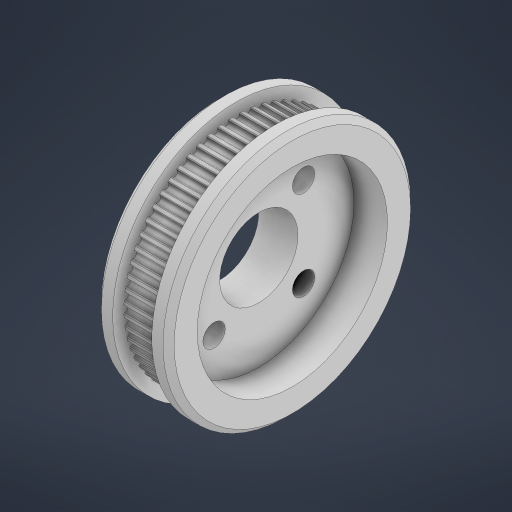
# Autodesk Inventor part: GT2 Pulley
Saved by Autodesk Inventor 2024 (Build 280153000, 153)
## iProperties
Created: 2023-10-25
Part Number: GT2 Pulley
Material: Generic
Document SubType Name: Modeling
Designer: avsar
Density: 1 g/cm^3
Appearance: Default
Author: avsar
Autodesk Inventor part; units mm, degrees
ref_plane "YZ Plane" through (0, 0, 0) normal (1, 0, 0) x (0, 1, 0)
ref_plane "XZ Plane" through (0, 0, 0) normal (0, 1, 0) x (-1, 0, 0)
ref_plane "XY Plane" through (0, 0, 0) normal (0, 0, 1) x (1, 0, 0)
sketch "Sketch1" plane through (0, 0, 0) normal (1, 0, 0) x (0, 1, 0)
  circle A0 centre (0, 0) radius 20.1178 construction
  circle A1 centre (0, 0) radius 19.3678 construction
  line L0 (0, 0) -> (20.1178, 0) construction
  line L1 (0, 0) -> (0, -20.1178) construction
  circle A2 centre (19.9228, 0) radius 0.555 construction
  line L2 (0, 0) -> (20.021, -1.9719) construction
  circle A3 centre (19.8269, -1.9528) radius 0.555 construction
  circle A4 centre (19.9554, -0.7042) radius 0.15 construction
  circle A5 centre (19.9283, -1.2551) radius 0.15 construction
  arc A6 (19.3678, 0) -> (19.9485, -0.5544) centre (19.9228, 0) ccw
  arc A7 (20.1053, -0.7095) -> (19.9485, -0.5544) centre (19.9554, -0.7042) ccw
  arc A8 (20.0781, -1.2645) -> (20.1053, -0.7095) centre (0, 0) ccw
  arc A9 (19.9068, -1.4036) -> (20.0781, -1.2645) centre (19.9283, -1.2551) ccw
  arc A10 (19.9068, -1.4036) -> (19.2746, -1.8984) centre (19.8269, -1.9528) ccw
  arc A11 (19.2746, -1.8984) -> (19.3678, 0) centre (0, 0) ccw
  dimension "d0" = 40.2357
  dimension "d1" = -0.75
  dimension "d2" = 1.11
  dimension "d4" = 84.375
  dimension "d5" = 0.3
  constraints: 25 point on circle, 12 centre point, 8 equal radius, 8 tangent, 6 end point, 4 point on line, 1 coincident, 1 concentric, 1 horizontal, 1 perpendicular
  measures "d0" diameter of A0
  measures "d1" radial gap between concentric circles of A0 A1
  measures "d2" diameter of A2
  measures "d4" angle of L1 L2
  measures "d5" diameter of A4
extrude "Extrusion1" add sketch "Sketch1" along normal mid plane 7
pattern_circular "Circular Pattern1" count 64 over 360 about axis through (-10, 0, 0) along (1, 0, 0) of "Extrusion1"
sketch "Sketch2" plane through (0, 0, 0) normal (1, 0, 0) x (0, 1, 0)
  arc A0 (19.2746, 1.8984) -> (19.9068, 1.4036) centre (19.8269, 1.9528) ccw projected
  circle A1 centre (0, 0) radius 19.3678
  constraints: 1 coincident, 3 other
extrude "Extrusion2" add sketch "Sketch2" along normal mid plane 7
sketch "Sketch3" plane through (3.5, 0, 0) normal (1, 0, 0) x (0, 0, -1)
  circle A0 centre (0, 0) radius 20.1178 construction
  arc A1 (1.2645, 20.0781) -> (0.7095, 20.1053) centre (0, 0) ccw projected
  circle A2 centre (0, 0) radius 22.1178
  point P0 (0.9871, 20.0936)
  dimension "d13" = 2
  constraints: 1 centre point, 1 coincident, 1 point on circle, 3 other
extrude "Extrusion3" add sketch "Sketch3" along normal blind 3
sketch "Sketch4" plane through (-3.5, 0, 0) normal (-1, 0, 0) x (0, 0, 1)
  circle A0 centre (0, 0) radius 22.1178 projected
extrude "Extrusion4" add sketch "Sketch4" along normal blind 3
sketch "Sketch5" plane through (-6.5, 0, 0) normal (-1, 0, 0) x (0, 0, 1)
  circle A0 centre (-8, 8) radius 2
  circle A1 centre (-8, -8) radius 2
  circle A2 centre (8, -8) radius 2
  circle A3 centre (8, 8) radius 2
  circle A4 centre (0, 0) radius 7
  dimension "d18" = 4
  dimension "d19" = 8
  dimension "d20" = 8
  dimension "d23" = 360
  dimension "d25" = 14
  constraints: 5 centre point, 1 coincident, 9 other
  measures "d18" diameter of A0
  measures "d19" horizontal distance of point (0, 0) A0.centre
  measures "d20" horizontal distance of point (0, 0) A0.centre
  measures "d25" diameter of A4
extrude "Extrusion5" cut sketch "Sketch5" against normal through all
chamfer "Chamfer1" distance 1 angle 45 2 edges at (-6.5, 0, -22.1178) (6.5, 0, 22.1178)
sketch "Sketch6" plane through (6.5, 0, 0) normal (1, 0, 0) x (0, 0, -1)
  circle A0 centre (0, 0) radius 17
  dimension "d31" = 34
  constraints: 1 centre point, 1 coincident
  measures "d31" diameter of A0
extrude "Extrusion6" cut sketch "Sketch6" against normal blind 6
equation "\"d0\" = OD_"
equation "\"d1\" = H_"
equation "\"d2\" = BTD_"
equation "\"d4\" = TH_"
equation "\"d5\" = PTR_"
equation "\"d6\" = EX_"
equation "\"d11\" = EX_"
equation "\"U_\" = 0.254"
equation "\"H_\" = -0.75"
equation "\"P_\" = 2"
equation "\"BTD_\" = 1.11"
equation "\"PTR_\" = 0.3"
equation "\"EX_\" = 7"
equation "\"OD_\" = PD_ - 2 * U_"
equation "\"TH_\" = 84.375deg"
equation "\"PD_\" = 40.743665"
body "Solid1"
